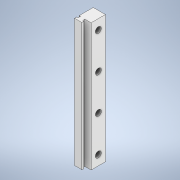
# Autodesk Inventor part: aactuatorHolder
Saved by Autodesk Inventor 2021 (Build 250183000, 183)
## iProperties
Created: 2021-03-21
Part Number: aactuatorHolder
Material: ABS Plastic
Document SubType Name: Modeling
Designer: Work
Mass: 34.0295 g
Surface Area: 123.061 cm^2
Volume: 32.1033 cm^3
Density: 1.06 g/cm^3
Appearance: Smooth - White
Author: Work
Autodesk Inventor part; units mm, degrees
ref_plane "YZ Plane" through (0, 0, 0) normal (1, 0, 0) x (0, 1, 0)
ref_plane "XZ Plane" through (0, 0, 0) normal (0, 1, 0) x (-1, 0, 0)
ref_plane "XY Plane" through (0, 0, 0) normal (0, 0, 1) x (1, 0, 0)
sketch "Sketch1" plane through (0, 0, 0) normal (0, 1, 0) x (-1, 0, 0)
  line L0 (0, 0) -> (0, -2.5)
  line L1 (0, 0) -> (-8.2, 0)
  line L2 (-8.2, 0) -> (-8.2, -2.3)
  line L3 (-8.2, -2.3) -> (-6.7, -2.3)
  line L4 (0, -2.5) -> (-1.5, -2.5)
  line L5 (-1.5, -2.5) -> (-1.5, -5)
  line L6 (-6.7, -2.3) -> (-6.7, -4.8)
  line L7 (-6.7, -4.8) -> (-13.6, -4.8)
  line L8 (-13.6, -4.8) -> (-13.6, -20.8)
  line L9 (-1.5, -5) -> (0, -5)
  line L10 (-13.6, -20.8) -> (0, -20.8)
  line L11 (0, -20.8) -> (0, -5)
  dimension "d0" = 2.5
  dimension "d1" = 8.2
  dimension "d2" = 2.3
  dimension "d3" = 1.5
  dimension "d4" = 1.5
  dimension "d5" = 2.5
  dimension "d6" = 2.5
  dimension "d7" = 6.9
  dimension "d8" = 16
  constraints: 24 end point, 6 horizontal, 3 perpendicular, 3 vertical
  measures "d0" distance of L0.start L0.end
  measures "d1" distance of L0.start L1.end
  measures "d2" distance of L1.end L2.end
  measures "d3" distance of L2.end L3.end
  measures "d4" distance of L0.end L4.end
  measures "d5" distance of L4.end L5.end
  measures "d6" distance of L3.end L6.end
  measures "d7" distance of L6.end L7.end
  measures "d8" distance of L7.end L8.end
extrude "Extrusion1" add sketch "Sketch1" along normal blind 142
sketch "Sketch2" plane through (0, 0, -20.8) normal (-1, 0, 0) x (0, 0, 1)
  line L0 (0, 142) -> (15.8, 142) projected
  line L1 (0, 0) -> (15.8, 0) projected
  point P0 (20.8, 0)
  point P1 (8, 131)
  point P2 (8, 11)
  point P3 (7.9, 51)
  point P4 (7.9, 91)
  dimension "d11" = 11
  dimension "d12" = 11
  dimension "d13" = 40
  dimension "d14" = 40
  measures "d11" distance from line of L0 point (8, 131)
  measures "d12" distance from line of L1 point (8, 11)
  measures "d13" vertical distance of point (7.9, 91) point (8, 131)
  measures "d14" vertical distance of point (7.9, 51) point (8, 11)
hole "Hole1" at (0, 131, -12.8) at (0, 11, -12.8) at (0, 51, -12.9) at (0, 91, -12.9) direction (1, 0, 0) diameter 6.604 end through all counterbore diameter 10.9982 counterbore depth 5.9944 clearance for "Socket Head Cap Screw" size "M6" standard "Ansi Metric M Profile"
body "Solid1"
